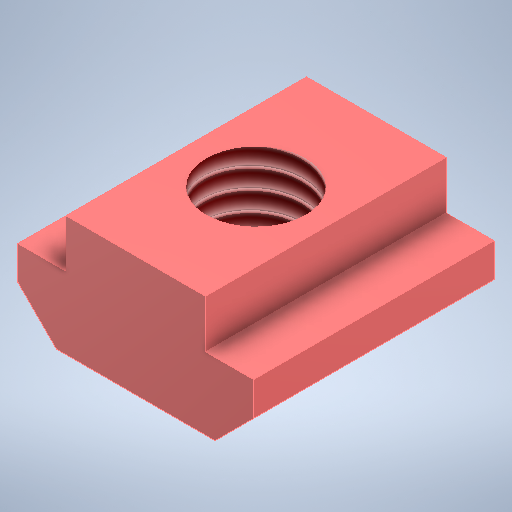
# Autodesk Inventor part: гайка T-паза m6
Saved by Autodesk Inventor 2025 (Build 290162000, 162)
## iProperties
Created: 2025-03-02
Part Number: гайка T-паза m6
Material: Типовые
Document SubType Name: Modeling
Designer: volko
Density: 1 g/cm^3
Appearance: Гладкий — красный
Categories: <MemberInstance><Categories><Category DisplayName="Крепежные изделия" InternalName="e4da775c-781d-43d5-af7c-5136215cf5a6" Mnemonic="FSTN"><Category DisplayName="Гайки" InternalName="e37c7a56-0470-4688-8db4-b4d75d611516" Mnemonic="NUT"><CategoryParameter DisplayName="Обозначение резьбы" InternalName="10aefdba-3783-44b8-becc-0feae870ab73" Mnemonic="thrdesign"/><CategoryParameter DisplayName="Обозначение серии резьб" InternalName="17a0ae10-6923-48a9-85c7-ae9b76790e6f" Mnemonic="thrserdsgn"/><CategoryParameter DisplayName="Тип резьбы" InternalName="205c6614-02f1-43b1-b704-b331415a8186" Mnemonic="thrtype"/><CategoryParameter DisplayName="Обозначение номинального диаметра" InternalName="39406bc0-754a-4a9f-8c64-e1bba9d40b8a" Mnemonic="nomdiadesig"/><CategoryParameter DisplayName="Высота" InternalName="5579c84d-d692-41f2-8996-171d03c19b53" Mnemonic="nheig"/><CategoryParameter DisplayName="Класс резьбы" InternalName="9b95427d-7bb5-461a-8a3e-4650073a592b" Mnemonic="thrclss"/><CategoryParameter DisplayName="Шаг резьбы" InternalName="bd2c58b1-df6d-45e3-8bf7-4a0997b15b95" Mnemonic="pitch1"/><CategoryParameter DisplayName="Номинальный диаметр" InternalName="d6e3b243-37ab-4432-98ea-592d296d3a46" Mnemonic="nomdia"/><CategoryParameter DisplayName="Витков на единицу" InternalName="e2e4d09d-bc7f-4af6-8086-8693b8d97bcd" Mnemonic="thrperunit1"/><Category DisplayName="Барашки" InternalName="f9aa88e7-8de7-4cd3-b433-3a5e01b39e94" Mnemonic="WNGNUT"><CategoryParameter DisplayName="Ширина по плоскостям" InternalName="57a06727-04fa-4a41-b524-e0f4b4ec340b" Mnemonic="waflat"/></Category></Category></Category></Categories><FamilyTemplate Id="гайка T-паза m6"><FamilyTemplateParameters/></FamilyTemplate><CategoryParameterMap><ParamToTemplateMap><ParamToTemplate CategoryParameter="//CategoryParameter[@InternalName='9b95427d-7bb5-461a-8a3e-4650073a592b']" ConstantValue="Отверстие1:Class"/><ParamToTemplate CategoryParameter="//CategoryParameter[@InternalName='10aefdba-3783-44b8-becc-0feae870ab73']" ConstantValue="Отверстие1:Designation"/><ParamToTemplate CategoryParameter="//CategoryParameter[@InternalName='205c6614-02f1-43b1-b704-b331415a8186']" ConstantValue="Отверстие1:Type"/><ParamToTemplate CategoryParameter="//CategoryParameter[@InternalName='bd2c58b1-df6d-45e3-8bf7-4a0997b15b95']" ConstantValue="Отверстие1:Pitch"/></ParamToTemplateMap></CategoryParameterMap></MemberInstance>
Author: volko
Autodesk Inventor part; units mm, degrees
ref_plane "YZ Plane" through (0, 0, 0) normal (1, 0, 0) x (0, 1, 0)
ref_plane "XZ Plane" through (0, 0, 0) normal (0, 1, 0) x (-1, 0, 0)
ref_plane "XY Plane" through (0, 0, 0) normal (0, 0, 1) x (1, 0, 0)
sketch "Эскиз2" plane through (0, 0, 0) normal (0, 0, 1) x (1, 0, 0)
  line L0 (-4.9, 3) -> (-4.9, 1.6)
  line L1 (-4.9, 1.6) -> (-3.3, 0)
  line L2 (-3.3, 0) -> (0, 0)
  line L3 (-4.9, 3) -> (-2.9, 3)
  line L4 (-2.9, 3) -> (-2.9, 5)
  line L5 (-2.9, 5) -> (0, 5)
  line L6 (-6.86, 0) -> (6.86, 0) projected
  line L7 (0, -1) -> (0, 6) projected
  line L8 (4.9, 3) -> (4.9, 1.6)
  line L9 (4.9, 1.6) -> (3.3, 0)
  line L10 (3.3, 0) -> (0, 0)
  line L11 (4.9, 3) -> (2.9, 3)
  line L12 (2.9, 3) -> (2.9, 5)
  line L13 (2.9, 5) -> (0, 5)
  point P0 (3.3, 0)
  dimension "d0" = 2
  dimension "d1" = 1.4
  dimension "d3" = 9.8
  dimension "d4" = 5.8
  dimension "d5" = 5
  dimension "d18" = 6.6
  constraints: 24 end point, 5 symmetric about line, 3 perpendicular, 1 horizontal, 1 point on line, 1 vertical
  measures "d0" distance between parallel lines of L3 L5
  measures "d1" distance of L0.start L0.end
  measures "d3" distance between parallel lines of L8 L0
  measures "d4" distance between parallel lines of L12 L4
  measures "d5" distance between parallel lines of L2 L5
  measures "d18" distance of L9.end L1.end
extrude "Выдавливание1" add sketch "Эскиз2" along normal mid plane 10
sketch "Эскиз3" plane through (-2.9, 5, 5) normal (0, 1, 0) x (1, 0, 0)
  point P0 (2.9, 5)
  point P1 (2.9, 5)
  constraints: 1 coincident
hole "Отверстие1" at (0, 5, 0) direction (0, -1, 0) diameter 4.134 end through all thread size "M5x0.8" class "6H" standard "ISO Metric profile"
